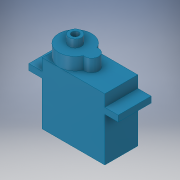
# Autodesk Inventor part: servo body
Saved by Autodesk Inventor 2017 (Build 210142000, 142)
## iProperties
Created: 2016-11-17
Part Number: servo body
Material: Generic
Document SubType Name: Modeling
Designer: PLTW
Density: 1 g/cm^3
Appearance: Sky Blue Dark
Author: PLTW
Autodesk Inventor part; units mm, degrees
ref_plane "YZ Plane" through (0, 0, 0) normal (1, 0, 0) x (0, 1, 0)
ref_plane "XZ Plane" through (0, 0, 0) normal (0, 1, 0) x (-1, 0, 0)
ref_plane "XY Plane" through (0, 0, 0) normal (0, 0, 1) x (1, 0, 0)
sketch "Sketch1" plane through (0, 0, 0) normal (0, 0, 1) x (1, 0, 0)
  line L0 (0, 0) -> (22.7838, 0)
  line L1 (22.7838, 0) -> (22.7838, 22.479)
  line L2 (22.7838, 22.479) -> (0, 22.479)
  line L3 (0, 22.479) -> (0, 0)
  dimension "d0" = 22.7838
  dimension "d1" = 22.479
  constraints: 8 end point, 2 parallel, 1 horizontal, 1 perpendicular
  measures "d0" distance of L1.end L2.end
  measures "d1" distance of L0.end L1.end
extrude "Extrusion1" add sketch "Sketch1" along normal blind 11.9888
sketch "Sketch2" plane through (0, 0, 0) normal (-1, 0, 0) x (0, 0, 1)
  line L0 (0, 22.479) -> (11.9888, 22.479) projected
  line L1 (0, 22.479) -> (0, 0) projected
  line L2 (0, 0) -> (11.9888, 0) projected
  line L3 (11.9888, 22.479) -> (11.9888, 0) projected
  line L4 (0, 22.479) -> (11.9888, 22.479) projected
  line L5 (0, 0) -> (0, 22.479) projected
  line L6 (11.9888, 0) -> (11.9888, 22.479) projected
  line L7 (0, 18.1864) -> (11.9888, 18.1864)
  line L8 (11.9888, 18.1864) -> (11.9888, 15.9766)
  line L9 (11.9888, 15.9766) -> (0, 15.9766)
  line L10 (0, 15.9766) -> (0, 18.1864)
  dimension "d4" = 2.2098
  dimension "d5" = 4.2926
  constraints: 8 end point, 2 parallel, 2 point on line, 1 horizontal, 1 perpendicular
  measures "d4" distance between parallel lines of L9 L7
  measures "d5" distance between parallel lines of L7 L0
extrude "Extrusion2" add sketch "Sketch2" along normal blind 4.8768 and the other way blind 27.6606 contours L7 L3 L9 L1
sketch "Sketch3" plane through (0, 0, 0) normal (-1, 0, 0) x (0, 0, 1)
  line L0 (0, 15.9766) -> (0, 0) projected
  line L1 (0, 0) -> (11.9888, 0) projected
  line L2 (4.2672, 5.715) -> (7.7216, 5.715)
  line L3 (7.7216, 5.715) -> (7.7216, 4.6228)
  line L4 (7.7216, 4.6228) -> (4.2672, 4.6228)
  line L5 (4.2672, 4.6228) -> (4.2672, 5.715)
  dimension "d10" = 3.4544
  dimension "d11" = 1.0922
  dimension "d12" = 4.6228
  dimension "d13" = 4.2672
  constraints: 8 end point, 2 parallel, 1 horizontal, 1 perpendicular
  measures "d10" distance of L2.start L2.end
  measures "d11" distance of L2.end L3.end
  measures "d12" distance between parallel lines of L1 L4
  measures "d13" distance between parallel lines of L0 L5
extrude "Extrusion3" add sketch "Sketch3" along normal blind 2.54
sketch "Sketch4" plane through (0, 22.479, 0) normal (0, 1, 0) x (1, 0, 0)
  line L0 (22.7838, 0) -> (0, 0) projected
  line L1 (0, 0) -> (0, -11.9888) projected
  line L2 (22.7838, -11.9888) -> (0, -11.9888) projected
  circle A0 centre (5.9944, -5.9944) radius 5.9944
  circle A1 centre (11.9888, -5.9944) radius 2.54
  dimension "d17" = 5.08
  constraints: 2 horizontal, 2 horizontal alignment, 1 centre point, 1 vertical, 2 other
  measures "d17" diameter of A1
extrude "Extrusion4" add sketch "Sketch4" along normal blind 4.6228 contours A0 A1 | A1 A0 | A0 A1
sketch "Sketch5" plane through (0, 27.1018, 0) normal (0, 1, 0) x (1, 0, 0)
  arc A0 (11.4507, -3.5121) -> (11.4507, -8.4767) centre (5.9944, -5.9944) ccw projected
  circle A1 centre (5.9944, -5.9944) radius 2.2606
  circle A2 centre (5.9944, -5.9944) radius 1.2827
  point P0 (0, 0)
  dimension "d20" = 4.5212
  dimension "d21" = 2.5654
  constraints: 2 centre point, 2 coincident
  measures "d20" diameter of A1
  measures "d21" diameter of A2
extrude "Extrusion5" add sketch "Sketch5" along normal blind 2.8448
body "Solid1"
